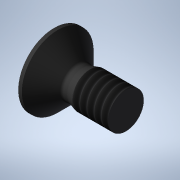
# Autodesk Inventor part: BFBJ2-4
Saved by Autodesk Inventor 2021 (Build 250183000, 183)
## iProperties
Created: 2025-06-03
Part Number: BFBJ2-4
Material: Generic
Catalog Web Link: www.cadenas.de
Description: BFBJ, SFBJ-Cross Recessed Flat Head Machine Screws
Vendor: MISUMI
Document SubType Name: Modeling
Designer: psAdmin
Manufacturer: MISUMI
Mass: 0.0169311 g
Surface Area: 0.539608 cm^2
Volume: 0.0169311 cm^3
Density: 1 g/cm^3
Appearance: PSOLRGB-175-175-175
Category: PARTsolutions
Company: MISUMI
Title: BFBJ2-4
Author: Cadenas PARTsolutions
Comments: Cross Recessed Flat Head Machine Screws
PSOL_IDENT_0: {$CADENAS_DATA/23d-libs/misumi/metric/27_screws_nuts/sfbj.prj},164 {VTYP=3D},{NB=BFBJ2-4},{LINA=BFBJ
PSOL_IDENT_1: 2-4},{NN=BFBJ, SFBJ},{DATE=29.11.2024 04:24:31},{GEOMDATE=15.12.2011 00:00:00},{VERSION=},{LINEID=10
PSOL_IDENT_2: },{WBVAR=MAT,L},{WBNUMERIC=L}  {NB=BFBJ2-4},{LINA=BFBJ2-4},{KT=DUMMY},{PN=BFBJ2-4},{TYPE=BFBJ},{MAT=
PSOL_IDENT_3: SWCH},{MATA='SWCH','SWCH Carbon Steel','SUS304','304 Stainless Steel'},{M=2},{M1=2.0},{L=4},{LA=3,4,
PSOL_IDENT_4: 5,6,8},{P=0.40},{MP=2x0.4},{A=4.0},{E=1.20},{MM=2.200},{CC=0.200},{RR=0.200}
NB: BFBJ2-4
NN: BFBJ, SFBJ
NT: Cross Recessed Flat Head Machine Screws
NBSYN: $PN.
LINA: BFBJ2-4
CATALOG: Misumi
PN: BFBJ2-4
MAT: SWCH Carbon Steel
M: 2
L: 4
MP: 2x0.4
A: 4
E: 1.2
SUPPLIER: MISUMI
ARTICLENO: BFBJ2-4
BOMINFO: BFBJ2-4
CREATOR: CADENAS GmbH
Autodesk Inventor part; units mm, degrees
sketch "Sketch_1" plane through (0, 0, 0) normal (0, 0, 1) x (1, 0, 0)
  line L0 (2.8, 0) -> (-1.2, 0)
  line L1 (-1.2, 0) -> (-1.2, 2)
  line L2 (-1.2, 2) -> (-1, 2)
  line L3 (-1, 2) -> (0.0642, 0.9358)
  arc A0 (0.0642, 0.9358) -> (0.2056, 0.8772) centre (0.2056, 1.0772) ccw
  line L4 (0.2056, 0.8772) -> (0.4, 0.8772)
  line L5 (0.4, 0.8772) -> (0.8, 1)
  line L6 (0.8, 1) -> (2.8, 1)
  line L7 (2.8, 1) -> (2.8, 0)
  line L8 (2.8, 0) -> (-1.2, 0)
  constraints: 18 end point, 2 point on circle, 1 centre point
revolve "Revolution1" add sketch "Sketch_1" angle 360 about axis through (2.8, 0, 0) along (1, 0, 0)
thread "Thread1" size "M2x0.4" class "6g" standard "ISO Metric profile" full length
sketch "Sketch_2" plane through (-1.2, 0, 0) normal (1, 0, 0) x (0, 0, -1)
  line L0 (-1.1, -0.2667) -> (-0.6667, -0.2667)
  arc A0 (-0.2667, -0.6667) -> (-0.6667, -0.2667) centre (-0.6667, -0.6667) ccw
  line L1 (-0.2667, -0.6667) -> (-0.2667, -1.1)
  line L2 (-0.2667, -1.1) -> (0.2667, -1.1)
  line L3 (0.2667, -1.1) -> (0.2667, -0.6667)
  arc A1 (0.6667, -0.2667) -> (0.2667, -0.6667) centre (0.6667, -0.6667) ccw
  line L4 (0.6667, -0.2667) -> (1.1, -0.2667)
  line L5 (1.1, -0.2667) -> (1.1, 0.2667)
  line L6 (1.1, 0.2667) -> (0.6667, 0.2667)
  arc A2 (0.2667, 0.6667) -> (0.6667, 0.2667) centre (0.6667, 0.6667) ccw
  line L7 (0.2667, 0.6667) -> (0.2667, 1.1)
  line L8 (0.2667, 1.1) -> (-0.2667, 1.1)
  line L9 (-0.2667, 1.1) -> (-0.2667, 0.6667)
  arc A3 (-0.6667, 0.2667) -> (-0.2667, 0.6667) centre (-0.6667, 0.6667) ccw
  line L10 (-0.6667, 0.2667) -> (-1.1, 0.2667)
  line L11 (-1.1, 0.2667) -> (-1.1, -0.2667)
  constraints: 24 end point, 8 point on circle, 4 centre point
extrude "Extrusion1" cut sketch "Sketch_2" along normal blind 0.6
ref_plane "bolt_XY" through (-1.2, 0, 0) normal (1, 0, 0) x (0, 0, -1)
ref_plane "bolt_YZ" through (-1.2, 0, 0) normal (0, 0, -1) x (0, 1, 0)
ref_plane "bolt_ZX" through (-1.2, 0, 0) normal (0, 1, 0) x (1, 0, 0)
ref_plane "nut_XY" through (2.8, 0, 0) normal (1, 0, 0) x (0, 0, -1)
ref_plane "nut_YZ" through (2.8, 0, 0) normal (0, 0, -1) x (0, 1, 0)
ref_plane "nut_ZX" through (2.8, 0, 0) normal (0, 1, 0) x (1, 0, 0)
body "Solid1"
